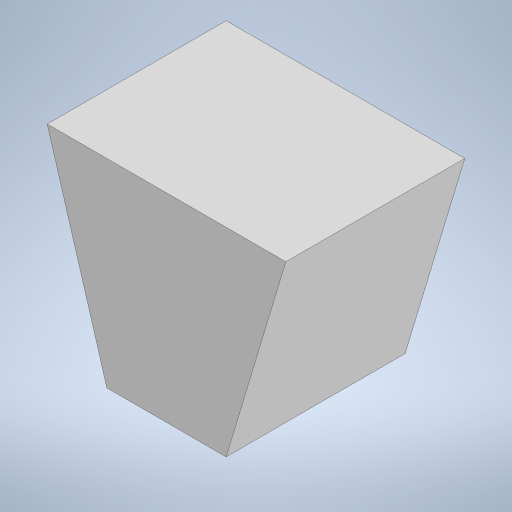
# Autodesk Inventor part: Trap
Saved by Autodesk Inventor 2024 (Build 280153000, 153)
## iProperties
Created: 2024-09-13
Part Number: Trap
Material: Generic
Document SubType Name: Modeling
Designer: srira
Density: 1 g/cm^3
Appearance: Default
Author: srira
Autodesk Inventor part; units mm, degrees
ref_plane "YZ Plane" through (0, 0, 0) normal (1, 0, 0) x (0, 1, 0)
ref_plane "XZ Plane" through (0, 0, 0) normal (0, 1, 0) x (-1, 0, 0)
ref_plane "XY Plane" through (0, 0, 0) normal (0, 0, 1) x (1, 0, 0)
sketch "Sketch1" plane through (0, 0, 0) normal (0, 0, 1) x (1, 0, 0)
  line L0 (-600, 0) -> (-595, 0)
  line L1 (-300, -1000) -> (-600, 0)
  line L2 (-300, -1000) -> (-295, -1000)
  line L3 (-295, -1000) -> (0, -1000)
  line L4 (-295, -995) -> (-295, -995.4434)
  line L5 (-595, 0) -> (-295, -995)
  line L6 (-295, -995) -> (0, -995)
  line L7 (0, -455.1044) -> (0, -112.5213) construction
  line L8 (600, 0) -> (595, 0)
  line L9 (300, -1000) -> (600, 0)
  line L10 (295, -1000) -> (0, -1000)
  line L11 (595, 0) -> (295, -995)
  line L12 (295, -995) -> (0, -995)
  line L13 (300, -1000) -> (295, -1000)
  point P0 (0, 0)
  dimension "d0" = 5
  dimension "d1" = 5
  dimension "d2" = 295
  constraints: 28 end point, 5 symmetric about line, 4 horizontal, 1 vertical
  measures "d0" distance of L0.start L0.end
  measures "d1" distance of L1.start L2.end
  measures "d2" distance of L2.end L3.end
extrude "Extrusion1" add sketch "Sketch1" along normal blind 900
sketch "Sketch2" plane through (0, 0, 900) normal (0, 0, 1) x (1, 0, 0)
  line L0 (-295, -995) -> (-595, 0) projected
  line L1 (-595, 0) -> (-295, -995)
  line L2 (-295, -995) -> (295, -995)
  line L3 (595, 0) -> (295, -995) projected
  line L4 (295, -995) -> (595, 0)
  line L5 (595, 0) -> (-595, 0)
  point P0 (0, 0)
  constraints: 8 end point, 2 collinear, 1 horizontal, 1 parallel
extrude "Extrusion2" add sketch "Sketch2" against normal blind 900
body "Solid1"
